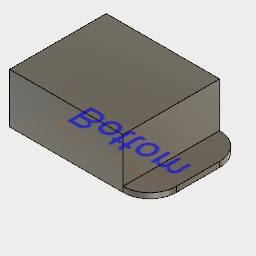
power brik v1 (Autodesk Fusion 360 design; units mm, degrees)
Autodesk Fusion 360 part; units mm, degrees
sketch "Sketch1" plane through (0, 0, 0) normal (0, 0, 1) x (1, 0, 0)
  line L0 (21, 14.5) -> (-21, 14.5)
  line L1 (-21, 14.5) -> (-21, -14.5)
  line L2 (-21, -14.5) -> (21, -14.5)
  line L3 (21, -14.5) -> (21, 14.5)
  line L4 (21, 14.5) -> (-21, -14.5) construction
  line L5 (-21, 14.5) -> (21, -14.5) construction
  dimension "d1" = 42
  dimension "d2" = 29
  measures "d1" distance of L1.end L2.end
  measures "d2" distance of L0.end L1.end
extrude "Extrude1" add sketch "Sketch1" along normal blind 15
fillet "Fillet1" radius 8 2 edges at (21, -14.5, 7.5) (21, 14.5, 7.5)
sketch "Sketch2" plane through (0, 0, 0) normal (0, 0, -1) x (1, 0, 0)
  arc A0 (13, -14.5) -> (21, -6.5) centre (13, -6.5) ccw
  line L0 (21, -6.5) -> (21, 6.5)
  arc A1 (21, 6.5) -> (13, 14.5) centre (13, 6.5) ccw
  line L1 (13, 14.5) -> (-21, 14.5)
  line L2 (-21, 14.5) -> (-21, -14.5)
  line L3 (-21, -14.5) -> (13, -14.5)
  line L4 (-21, -14.5) -> (-11, -14.5)
  line L5 (-11, -14.5) -> (-11, -4.5)
  line L6 (-11, -4.5) -> (-21, -4.5)
  line L7 (-21, -4.5) -> (-21, -14.5)
  dimension "d6" = 10
  dimension "d7" = 10
  measures "d6" distance of L5.end L6.end
  measures "d7" distance of L4.end L5.end
extrude "Extrude2" add sketch "Sketch2" along normal blind 9 contours L2 L3 L4 L5 L6 L7
sketch "Sketch3" plane through (0, 0, 0) normal (0, 0, -1) x (1, 0, 0)
  line L0 (-11, -4.5) -> (-11, -14.5)
  line L1 (-11, -14.5) -> (13, -14.5)
  arc A0 (13, -14.5) -> (21, -6.5) centre (13, -6.5) ccw
  line L2 (21, -6.5) -> (21, 6.5)
  arc A1 (21, 6.5) -> (13, 14.5) centre (13, 6.5) ccw
  line L3 (13, 14.5) -> (-21, 14.5)
  line L4 (-21, 14.5) -> (-21, -4.5)
  line L5 (-21, -4.5) -> (-11, -4.5)
  line L6 (-14.2092, -3.0986) -> (16.0935, -3.0986) construction
  line L7 (16.0935, -3.0986) -> (16.0935, 6.9014) construction
  line L8 (16.0935, 6.9014) -> (-14.2092, 6.9014) construction
  line L9 (-14.2092, 6.9014) -> (-14.2092, -3.0986) construction
sketch "Sketch4" plane through (0, 0, 15) normal (0, 0, 1) x (-1, 0, 0)
  arc A0 (-21, -6.5) -> (-13, -14.5) centre (-13, -6.5) ccw
  line L0 (-13, -14.5) -> (21, -14.5)
  line L1 (21, -14.5) -> (21, 14.5)
  line L2 (21, 14.5) -> (-13, 14.5)
  arc A1 (-13, 14.5) -> (-21, 6.5) centre (-13, 6.5) ccw
  line L3 (-21, 6.5) -> (-21, -6.5)
  line L4 (-13, 14.5) -> (-29, 14.5)
  line L5 (-29, 14.5) -> (-29, -20)
  line L6 (-29, -20) -> (-13, -20)
  line L7 (-13, -20) -> (-13, 14.5)
extrude "Extrude3" cut sketch "Sketch4" against normal blind 13.4 contours A0 A1 L3 L7 | A0 A1 L3 L4 L5 L6 L7
equation "d10 = -15 mm + 1.6 mm"
